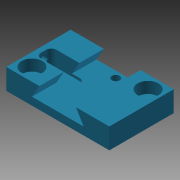
# Autodesk Inventor part: 13_1087_032
Saved by Autodesk Inventor 2014 SP1 (Build 180222100, 222)
## iProperties
Created: 2013-05-21
Part Number: 13_1087_032
Material: Allgemein
Document SubType Name: Modeling
Designer: vogel
Density: 1 g/cm^3
Appearance: Türkis
Author: vogel
Autodesk Inventor part; units mm, degrees
ref_plane "YZ Plane" through (0, 0, 0) normal (1, 0, 0) x (0, 1, 0)
ref_plane "XZ Plane" through (0, 0, 0) normal (0, 1, 0) x (-1, 0, 0)
ref_plane "XY Plane" through (0, 0, 0) normal (0, 0, 1) x (1, 0, 0)
sketch "Skizze1" plane through (0, 0, 0) normal (0, 0, 1) x (1, 0, 0)
  line L0 (-20, 12.5) -> (20, 12.5)
  line L1 (20, 12.5) -> (20, -12.5)
  line L2 (20, -12.5) -> (-20, -12.5)
  line L3 (-20, -12.5) -> (-20, 12.5)
  line L4 (-28, 0) -> (28, 0) projected
  line L5 (0, -17.5) -> (0, 17.5) projected
  point P0 (0, 0)
  dimension "d0" = 40
  dimension "d1" = 25
  constraints: 8 end point, 2 parallel, 1 horizontal, 1 perpendicular, 2 other
  measures "d0" distance of L0.start L0.end
  measures "d1" distance of L2.end L0.start
extrude "Extrusion1" add sketch "Skizze1" along normal blind 8
sketch "Skizze2" plane through (0, 0, 8) normal (0, 0, 1) x (1, 0, 0)
  line L0 (-28, 0) -> (28, 0) projected
  line L1 (0, -17.5) -> (0, 17.5) projected
  line L2 (-15, 7.5) -> (15, 7.5)
  line L3 (15, 7.5) -> (15, -7.5)
  line L4 (15, -7.5) -> (-15, -7.5)
  line L5 (-15, -7.5) -> (-15, 7.5)
  point P0 (0, 0)
  dimension "d4" = 15
  dimension "d5" = 30
  constraints: 8 end point, 2 coincident, 2 parallel, 1 horizontal, 1 perpendicular, 2 other
  measures "d4" distance of L4.end L2.start
  measures "d5" distance of L2.start L2.end
hole "Bohrung1" at (-15, -7.5, 8) at (15, 7.5, 8) direction (0, 0, -1) diameter 4.5 end through all counterbore diameter 8 counterbore depth 4.4
sketch "Skizze5" plane through (-20, -12.5, 0) normal (0, -1, 0) x (1, 0, 0)
  line L0 (40, 8) -> (0, 8) projected
  line L1 (-8, 0) -> (48, 0) projected
  line L2 (20, -1.6) -> (20, 9.6) projected
  line L3 (12.8868, 8) -> (27.1132, 8)
  line L4 (27.1132, 8) -> (30, 3)
  line L5 (30, 3) -> (10, 3)
  line L6 (10, 3) -> (12.8868, 8)
  point P0 (20, 0)
  dimension "d37" = 5
  dimension "d38" = 60
  dimension "d39" = 20
  constraints: 8 end point, 2 point on line, 1 parallel, 1 other
  measures "d37" distance between parallel lines of L5 L0
  measures "d38" angle of L6 L5
  measures "d39" distance of L4.end L5.end
extrude "Extrusion2" cut sketch "Skizze5" against normal through all
sketch "Skizze6" plane through (0, 0, 0) normal (0, 0, -1) x (-1, 0, 0)
  line L0 (28, 0) -> (-28, 0) projected
  line L1 (0, -17.5) -> (0, 17.5) projected
  point P0 (0, 0)
  point P1 (0, 10)
  dimension "d42" = 10
  constraints: 1 point on line
  measures "d42" distance from line of L0 point (0, 10)
hole "Bohrung5" at (0, 10, 0) direction (0, 0, 1) diameter 3 end through all
sketch "Skizze7" plane through (0, 0, 8) normal (0, 0, 1) x (1, 0, 0)
  line L0 (-20, -12.5) -> (-20, 12.5) projected
  line L1 (-28, 0) -> (28, 0) projected
  line L2 (0, -17.5) -> (0, 17.5) projected
  line L3 (-16, 3) -> (-7, 3)
  line L4 (-5, 1) -> (-5, -1)
  line L5 (-7, -3) -> (-16, -3)
  line L6 (-18, -1) -> (-18, 1)
  arc A0 (-16, 3) -> (-18, 1) centre (-16, 1) ccw
  arc A1 (-18, -1) -> (-16, -3) centre (-16, -1) ccw
  arc A2 (-7, -3) -> (-5, -1) centre (-7, -1) ccw
  arc A3 (-5, 1) -> (-7, 3) centre (-7, 1) ccw
  point P0 (0, 0)
  dimension "d53" = 2
  dimension "d54" = 15
  dimension "d55" = 13
  dimension "d56" = 2
  dimension "d57" = 6
  constraints: 8 end point, 8 point on circle, 8 tangent, 4 centre point, 3 equal radius, 2 parallel, 1 horizontal, 1 perpendicular, 1 other
  measures "d53" radius of A0
  measures "d54" distance between parallel lines of L4 L0
  measures "d55" distance between parallel lines of L4 L6
  measures "d56" radius of A3
  measures "d57" distance between parallel lines of L5 L3
extrude "Extrusion3" cut sketch "Skizze7" against normal blind 6
sketch "Skizze8" plane through (-20, -12.5, 0) normal (-1, 0, 0) x (0, 0, 1)
  line L0 (8, 0) -> (8, 25) projected
  line L1 (8, 15.5) -> (3, 15.5) projected
  line L2 (8, 15.5) -> (2, 15.5) projected
  line L3 (3, 15.5) -> (2, 15.5) projected
  line L4 (3.6, 1) -> (3.6, 9) projected
  line L5 (3, 9.5) -> (2, 9.5) projected
  line L6 (8, 9.5) -> (2, 9.5) projected
  line L7 (3, 9.5) -> (8, 9.5) projected
  line L8 (0, -5) -> (0, 30) projected
  line L9 (-1.6, 12.5) -> (9.6, 12.5) projected
  point P0 (0, 12.5)
  point P1 (5, 12.5)
  dimension "d60" = 3
  constraints: 1 point on line
  measures "d60" distance from line of point (5, 12.5) L0
hole "Bohrung6" at (-20, 0, 5) direction (1, 0, 0) diameter 3 depth 3 tip angle 118
hole "Bohrung7" at (-20, 8.5, 4) direction (1, 0, 0) diameter 2.459 depth 8 tip angle 118 thread size "M3x0.5" class "6H" standard "ISO Metric profile"
